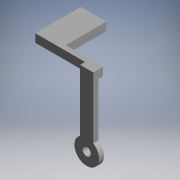
# Autodesk Inventor part: armV
Saved by Autodesk Inventor 2019 (Build 230136000, 136)
## iProperties
Created: 2020-04-01
Part Number: armV
Material: Generic
Document SubType Name: Modeling
Designer: Pulag
Density: 1 g/cm^3
Appearance: Default
Author: Pulag
Autodesk Inventor part; units mm, degrees
ref_plane "YZ Plane" through (0, 0, 0) normal (1, 0, 0) x (0, 1, 0)
ref_plane "XZ Plane" through (0, 0, 0) normal (0, 1, 0) x (-1, 0, 0)
sketch "Sketch1" plane through (0, 0, 0) normal (0, 0, 1) x (1, 0, 0)
  line L0 (6.9956, 3.6314) -> (6.4167, 3.8711) projected
  line L1 (5.7956, 3.9529) -> (6.4167, 3.8711) projected
  line L2 (5.1744, 3.8711) -> (5.7956, 3.9529) projected
  line L3 (4.5956, 3.6314) -> (5.1744, 3.8711) projected
  line L4 (4.0985, 3.25) -> (4.5956, 3.6314) projected
  line L5 (3.7171, 2.7529) -> (4.0985, 3.25) projected
  line L6 (3.4773, 2.1741) -> (3.7171, 2.7529) projected
  line L7 (3.4773, 2.1741) -> (3.3956, 1.5529) projected
  line L8 (3.4773, 0.9317) -> (3.3956, 1.5529) projected
  line L9 (3.4773, 0.9317) -> (3.7171, 0.3529) projected
  line L10 (3.7171, 0.3529) -> (4.0985, -0.1441) projected
  line L11 (4.0985, -0.1441) -> (4.5956, -0.5255) projected
  line L12 (4.5956, -0.5255) -> (5.1744, -0.7653) projected
  line L13 (5.1744, -0.7653) -> (5.7956, -0.8471) projected
  line L14 (5.7956, -0.8471) -> (6.4167, -0.7653) projected
  line L15 (6.4167, -0.7653) -> (6.9956, -0.5255) projected
  line L16 (6.9956, -0.5255) -> (7.4926, -0.1441) projected
  line L17 (7.4926, -0.1441) -> (7.874, 0.3529) projected
  line L18 (8.1138, 0.9317) -> (7.874, 0.3529) projected
  line L19 (8.1138, 0.9317) -> (8.1956, 1.5529) projected
  line L20 (8.1956, 1.5529) -> (8.1138, 2.1741) projected
  line L21 (8.1138, 2.1741) -> (7.874, 2.7529) projected
  line L22 (7.874, 2.7529) -> (7.4926, 3.25) projected
  line L23 (6.9956, 3.6314) -> (7.4926, 3.25) projected
  line L24 (6.7956, 1.5529) -> (6.7615, 1.8117) projected
  line L25 (6.7615, 1.2941) -> (6.7956, 1.5529) projected
  line L26 (6.6616, 1.0529) -> (6.7615, 1.2941) projected
  line L27 (6.5027, 0.8458) -> (6.6616, 1.0529) projected
  line L28 (6.2956, 0.6869) -> (6.5027, 0.8458) projected
  line L29 (6.0544, 0.587) -> (6.2956, 0.6869) projected
  line L30 (5.7956, 0.5529) -> (6.0544, 0.587) projected
  line L31 (5.5367, 0.587) -> (5.7956, 0.5529) projected
  line L32 (5.2956, 0.6869) -> (5.5367, 0.587) projected
  line L33 (5.0884, 0.8458) -> (5.2956, 0.6869) projected
  line L34 (4.9295, 1.0529) -> (5.0884, 0.8458) projected
  line L35 (4.8296, 1.2941) -> (4.9295, 1.0529) projected
  line L36 (4.7956, 1.5529) -> (4.8296, 1.2941) projected
  line L37 (4.7956, 1.5529) -> (4.8296, 1.8117) projected
  line L38 (4.8296, 1.8117) -> (4.9295, 2.0529) projected
  line L39 (4.9295, 2.0529) -> (5.0884, 2.26) projected
  line L40 (5.0884, 2.26) -> (5.2956, 2.4189) projected
  line L41 (5.2956, 2.4189) -> (5.5367, 2.5188) projected
  line L42 (5.5367, 2.5188) -> (5.7956, 2.5529) projected
  line L43 (5.7956, 2.5529) -> (6.0544, 2.5188) projected
  line L44 (6.0544, 2.5188) -> (6.2956, 2.4189) projected
  line L45 (6.2956, 2.4189) -> (6.5027, 2.26) projected
  line L46 (6.5027, 2.26) -> (6.6616, 2.0529) projected
  line L47 (6.6616, 2.0529) -> (6.7615, 1.8117) projected
  circle A0 centre (5.7956, 1.5529) radius 2.5
  arc A1 (1.7956, 7.8972) -> (9.7955, 7.8972) centre (5.7956, 1.5529) ccw
  line L48 (-28.4804, 55.5109) -> (-15.9804, 55.5109) projected
  line L49 (-28.4804, 55.5109) -> (-28.4804, 40.3109) projected
  line L50 (-15.9804, 40.3109) -> (-28.4804, 40.3109) projected
  line L51 (-15.9804, 40.3109) -> (-15.9804, 55.5109) projected
  line L52 (-20.6474, 51.7815) -> (-20.6304, 51.9109) projected
  line L53 (-20.6974, 51.6609) -> (-20.6474, 51.7815) projected
  line L54 (-20.7768, 51.5573) -> (-20.6974, 51.6609) projected
  line L55 (-20.8804, 51.4779) -> (-20.7768, 51.5573) projected
  line L56 (-21.001, 51.4279) -> (-20.8804, 51.4779) projected
  line L57 (-21.1304, 51.4109) -> (-21.001, 51.4279) projected
  line L58 (-21.2598, 51.4279) -> (-21.1304, 51.4109) projected
  line L59 (-21.3804, 51.4779) -> (-21.2598, 51.4279) projected
  line L60 (-21.4839, 51.5573) -> (-21.3804, 51.4779) projected
  line L61 (-21.5634, 51.6609) -> (-21.4839, 51.5573) projected
  line L62 (-21.5634, 51.6609) -> (-21.6133, 51.7815) projected
  line L63 (-21.6133, 51.7815) -> (-21.6304, 51.9109) projected
  line L64 (-21.6304, 51.9109) -> (-21.6133, 52.0403) projected
  line L65 (-21.5634, 52.1609) -> (-21.6133, 52.0403) projected
  line L66 (-21.4839, 52.2645) -> (-21.5634, 52.1609) projected
  line L67 (-21.3804, 52.3439) -> (-21.4839, 52.2645) projected
  line L68 (-21.3804, 52.3439) -> (-21.2598, 52.3939) projected
  line L69 (-21.2598, 52.3939) -> (-21.1304, 52.4109) projected
  line L70 (-21.1304, 52.4109) -> (-21.001, 52.3939) projected
  line L71 (-21.001, 52.3939) -> (-20.8804, 52.3439) projected
  line L72 (-20.8804, 52.3439) -> (-20.7768, 52.2645) projected
  line L73 (-20.7768, 52.2645) -> (-20.6974, 52.1609) projected
  line L74 (-20.6974, 52.1609) -> (-20.6474, 52.0403) projected
  line L75 (-20.6304, 51.9109) -> (-20.6474, 52.0403) projected
  line L76 (-21.7474, 51.7815) -> (-21.7304, 51.9109) projected
  line L77 (-21.7974, 51.6609) -> (-21.7474, 51.7815) projected
  line L78 (-21.8768, 51.5573) -> (-21.7974, 51.6609) projected
  line L79 (-21.9804, 51.4779) -> (-21.8768, 51.5573) projected
  line L80 (-22.101, 51.4279) -> (-21.9804, 51.4779) projected
  line L81 (-22.2304, 51.4109) -> (-22.101, 51.4279) projected
  line L82 (-22.3598, 51.4279) -> (-22.2304, 51.4109) projected
  line L83 (-22.4804, 51.4779) -> (-22.3598, 51.4279) projected
  line L84 (-22.5839, 51.5573) -> (-22.4804, 51.4779) projected
  line L85 (-22.6634, 51.6609) -> (-22.5839, 51.5573) projected
  line L86 (-22.6634, 51.6609) -> (-22.7133, 51.7815) projected
  line L87 (-22.7133, 51.7815) -> (-22.7304, 51.9109) projected
  line L88 (-22.7304, 51.9109) -> (-22.7133, 52.0403) projected
  line L89 (-22.6634, 52.1609) -> (-22.7133, 52.0403) projected
  line L90 (-22.5839, 52.2645) -> (-22.6634, 52.1609) projected
  line L91 (-22.4804, 52.3439) -> (-22.5839, 52.2645) projected
  line L92 (-22.4804, 52.3439) -> (-22.3598, 52.3939) projected
  line L93 (-22.3598, 52.3939) -> (-22.2304, 52.4109) projected
  line L94 (-22.2304, 52.4109) -> (-22.101, 52.3939) projected
  line L95 (-22.101, 52.3939) -> (-21.9804, 52.3439) projected
  line L96 (-21.9804, 52.3439) -> (-21.8768, 52.2645) projected
  line L97 (-21.8768, 52.2645) -> (-21.7974, 52.1609) projected
  line L98 (-21.7974, 52.1609) -> (-21.7474, 52.0403) projected
  line L99 (-21.7304, 51.9109) -> (-21.7474, 52.0403) projected
  line L100 (-22.8474, 51.7815) -> (-22.8304, 51.9109) projected
  line L101 (-22.8974, 51.6609) -> (-22.8474, 51.7815) projected
  line L102 (-22.9768, 51.5573) -> (-22.8974, 51.6609) projected
  line L103 (-23.0804, 51.4779) -> (-22.9768, 51.5573) projected
  line L104 (-23.201, 51.4279) -> (-23.0804, 51.4779) projected
  line L105 (-23.3304, 51.4109) -> (-23.201, 51.4279) projected
  line L106 (-23.4598, 51.4279) -> (-23.3304, 51.4109) projected
  line L107 (-23.5804, 51.4779) -> (-23.4598, 51.4279) projected
  line L108 (-23.6839, 51.5573) -> (-23.5804, 51.4779) projected
  line L109 (-23.7634, 51.6609) -> (-23.6839, 51.5573) projected
  line L110 (-23.7634, 51.6609) -> (-23.8133, 51.7815) projected
  line L111 (-23.8133, 51.7815) -> (-23.8304, 51.9109) projected
  line L112 (-23.8304, 51.9109) -> (-23.8133, 52.0403) projected
  line L113 (-23.7634, 52.1609) -> (-23.8133, 52.0403) projected
  line L114 (-23.6839, 52.2645) -> (-23.7634, 52.1609) projected
  line L115 (-23.5804, 52.3439) -> (-23.6839, 52.2645) projected
  line L116 (-23.5804, 52.3439) -> (-23.4598, 52.3939) projected
  line L117 (-23.4598, 52.3939) -> (-23.3304, 52.4109) projected
  line L118 (-23.3304, 52.4109) -> (-23.201, 52.3939) projected
  line L119 (-23.201, 52.3939) -> (-23.0804, 52.3439) projected
  line L120 (-23.0804, 52.3439) -> (-22.9768, 52.2645) projected
  line L121 (-22.9768, 52.2645) -> (-22.8974, 52.1609) projected
  line L122 (-22.8974, 52.1609) -> (-22.8474, 52.0403) projected
  line L123 (-22.8304, 51.9109) -> (-22.8474, 52.0403) projected
  line L124 (-21.6304, 37.8109) -> (-21.6304, 40.3109) projected
  line L125 (-15.9804, 37.8109) -> (-21.6304, 37.8109) projected
  line L126 (-15.9804, 37.8109) -> (-15.9804, 40.3109) projected
  line L127 (-21.6304, 40.3109) -> (-15.9804, 40.3109) projected
  line L128 (-28.4804, 37.8109) -> (-28.4804, 40.3109) projected
  line L129 (-22.8304, 37.8109) -> (-28.4804, 37.8109) projected
  line L130 (-22.8304, 37.8109) -> (-22.8304, 40.3109) projected
  line L131 (-28.4804, 40.3109) -> (-22.8304, 40.3109) projected
  line L132 (-28.4804, 40.3109) -> (-15.9804, 40.3109)
  line L133 (-15.9804, 40.3109) -> (-15.9804, 45.3109)
  line L134 (-15.9804, 45.3109) -> (-28.4804, 45.3109)
  line L135 (-28.4804, 45.3109) -> (-28.4804, 40.3109)
  line L136 (-15.9804, 45.3109) -> (-12.9804, 45.3109)
  line L137 (-12.9804, 45.3109) -> (-12.9804, 40.3109)
  line L138 (-12.9804, 40.3109) -> (-15.9804, 40.3109)
  line L139 (-15.9804, 40.3109) -> (-15.9804, 45.3109)
  line L140 (-28.4804, 45.3109) -> (-31.4804, 45.3109)
  line L141 (-31.4804, 45.3109) -> (-31.4804, 40.3109)
  line L142 (-31.4804, 40.3109) -> (-28.4804, 40.3109)
  line L143 (-28.4804, 40.3109) -> (-28.4804, 45.3109)
  line L144 (-12.9804, 45.3109) -> (5.7956, 45.3109)
  line L145 (1.7956, 40.3109) -> (-12.9804, 40.3109)
  line L146 (-12.9804, 40.3109) -> (-12.9804, 45.3109)
  line L147 (9.7956, 45.3109) -> (9.7955, 7.8972)
  line L148 (1.7956, 7.8972) -> (1.7956, 40.3109)
  line L149 (1.7956, 45.3109) -> (9.7956, 45.3109)
  line L150 (9.7956, 45.3109) -> (1.7956, 3.9529) construction
  line L151 (9.7956, 3.9529) -> (1.7956, 45.3109) construction
  line L152 (5.7956, 4.0529) -> (5.7956, 3.9529)
  line L153 (5.7956, 1.5529) -> (-36.8703, 1.5529)
  line L154 (-22.2304, 45.3109) -> (-22.2304, 1.5529)
  line L155 (1.7956, 39.0609) -> (1.7956, 45.3109)
  point P0 (0, 0)
  point P1 (5.7956, 24.6319)
  dimension "d0" = 5
  dimension "d1" = 15
  dimension "d2" = 5
  dimension "d3" = 3
  dimension "d4" = 3
  dimension "d6" = 8
  constraints: 48 end point, 9 parallel, 5 horizontal, 4 midpoint, 4 perpendicular, 4 point on line, 2 coincident, 2 point on circle, 1 centre point, 1 vertical, 3 other
  measures "d1" diameter of A1
  measures "d2" distance of L133.end L132.end
  measures "d3" distance of L137.end L138.end
  measures "d4" distance of L142.end L141.end
  measures "d6" distance of L151.start L150.end
extrude "Extrusion1" add sketch "Sketch1" along normal blind 3 contours A1 L148 L155 L144 L149 L147
sketch "Sketch2" plane through (1.7956, 39.0609, 0) normal (-1, 0, 0) x (0, 0, 1)
  line L0 (-5.2631, 16.45) -> (-5.2631, 1.25) projected
  line L1 (-27.7631, 1.25) -> (-27.7631, 16.45) projected
  line L2 (-5.2631, 16.45) -> (-27.7631, 16.45) projected
  line L3 (-27.7631, 1.25) -> (-27.7631, 16.45) projected
  line L4 (-27.7631, 1.25) -> (-32.5631, 1.25) projected
  line L5 (-32.5631, 1.25) -> (-32.5631, -1.25) projected
  line L6 (-27.7631, -1.25) -> (-32.5631, -1.25) projected
  line L7 (-27.7631, -1.25) -> (-27.7631, -5.75) projected
  line L8 (-5.2631, -5.75) -> (-27.7631, -5.75) projected
  line L9 (-5.2631, -1.25) -> (-5.2631, -5.75) projected
  line L10 (-5.2631, -1.25) -> (-0.4631, -1.25) projected
  line L11 (-0.4631, -1.25) -> (-0.4631, 1.25) projected
  line L12 (-5.2631, 1.25) -> (-0.4631, 1.25) projected
  line L13 (-5.2631, 16.45) -> (-5.2631, 1.25) projected
  line L14 (0, 6.25) -> (0, 0) projected
  line L15 (-27.7631, 1.25) -> (0, 1.25)
  line L16 (0, 1.25) -> (0, 6.25)
  line L17 (0, 6.25) -> (-27.7631, 6.25)
  line L18 (-27.7631, 6.25) -> (-27.7631, 1.25)
  line L19 (-27.7631, 6.25) -> (-30.7631, 6.25)
  line L20 (-30.7631, 6.25) -> (-30.7631, 1.25)
  line L21 (-30.7631, 1.25) -> (-27.7631, 1.25)
  line L22 (-27.7631, 1.25) -> (-27.7631, 6.25)
  point P0 (0, -39.0609)
  dimension "d9" = 3
  constraints: 16 end point, 4 parallel, 2 horizontal, 2 perpendicular, 1 point on line
  measures "d9" distance of L21.end L20.end
ref_plane "Work Plane1" through (-28.4804, 33.3109, -32.5631) normal (-1, 0, 0) x (0, 0, 1)
extrude "Extrusion2" add sketch "Sketch2" against normal blind 15.5 from surface at 30.276 contours L17 L14 L15 L12 L0 | L0 L15 L1 L17
sketch "Sketch3" plane through (-12.9804, 40.3109, 0) normal (1, 0, 0) x (0, 0, -1)
  line L0 (0, -32.4137) -> (0, 5) projected
  line L1 (0, 5) -> (-3, 5) projected
  line L2 (-3, -32.4137) -> (-3, 5) projected
  line L3 (0, -32.4137) -> (-3, -32.4137) projected
  line L4 (0, 5) -> (0, 0) projected
  line L5 (0, 0) -> (27.7631, 0) projected
  line L6 (27.7631, 0) -> (27.7631, 5) projected
  line L7 (27.7631, 5) -> (0, 5) projected
  line L8 (27.7631, 5) -> (0, 5) projected
  line L9 (0, 0) -> (3, 0)
  line L10 (3, 0) -> (3, 5)
  line L11 (3, 5) -> (0, 5)
  line L12 (0, 5) -> (0, 0)
  point P0 (0, -40.3109)
  dimension "d12" = 3
  constraints: 8 end point, 2 parallel, 1 horizontal, 1 perpendicular, 1 point on line
  measures "d12" distance of L11.end L10.end
extrude "Extrusion3" add sketch "Sketch3" along normal up to surface (22.776 mm away) contours L0 L7 L10 L5
body "Solid1"
